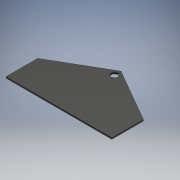
# Autodesk Inventor part: BA15
Saved by Autodesk Inventor 2017 (Build 210142000, 142)
## iProperties
Created: 2019-05-29
Part Number: BA15
Material: Wood (Cherry)
Document SubType Name: Modeling
Designer: Dell
Density: 0.63 g/cm^3
Appearance: Smooth - Black
Mass: 254.003 g
Surface Area: 1468.73 cm^2
Volume: 403.179 cm^3
Author: Dell
Autodesk Inventor part; units mm, degrees
ref_plane "YZ Plane" through (0, 0, 0) normal (1, 0, 0) x (0, 1, 0)
ref_plane "XZ Plane" through (0, 0, 0) normal (0, 1, 0) x (-1, 0, 0)
ref_plane "XY Plane" through (0, 0, 0) normal (0, 0, 1) x (1, 0, 0)
sketch "Sketch1" plane through (0, 0, 0) normal (0, 0, 1) x (1, 0, 0)
  line L0 (0, 0) -> (0, 201.9592)
  line L1 (0, 201.9592) -> (262.89, 353.7388)
  line L2 (262.89, 353.7388) -> (525.78, 201.9592)
  line L3 (525.78, 201.9592) -> (525.78, 0)
  line L4 (525.78, 0) -> (0, 0)
  point P0 (262.89, 0)
  dimension "d0" = 525.78
  dimension "d1" = 120
  dimension "d2" = 201.9592
  constraints: 10 end point, 1 horizontal alignment, 1 midpoint, 1 parallel, 1 perpendicular, 1 vertical, 1 vertical alignment
  measures "d0" distance of L3.end L0.start
  measures "d1" angle of L2 L1
  measures "d2" distance of L0.start L0.end
extrude "Extrusion1" add sketch "Sketch1" along normal blind 6.35
sketch "Sketch3" plane through (0, 0, 6.35) normal (0, 0, 1) x (1, 0, 0)
  line L0 (50.8, 180.4886) -> (474.98, 180.4886)
  line L1 (474.98, 180.4886) -> (474.98, 50.8)
  line L2 (474.98, 50.8) -> (50.8, 50.8)
  line L3 (50.8, 50.8) -> (50.8, 180.4886)
  line L4 (0, 201.9592) -> (0, 0) projected
  line L5 (50.8, 180.4886) -> (262.89, 302.9388)
  line L6 (262.89, 302.9388) -> (474.98, 180.4886)
  line L7 (525.78, 0) -> (0, 0) projected
  line L8 (0, 201.9592) -> (0, 0) projected
  line L9 (0, 0) -> (525.78, 0) projected
  line L10 (525.78, 0) -> (525.78, 201.9592) projected
  line L11 (525.78, 201.9592) -> (262.89, 353.7388) projected
  line L12 (262.89, 353.7388) -> (0, 201.9592) projected
  point P0 (262.89, 180.4886)
  dimension "d15" = 120
  dimension "d16" = 50.8
  dimension "d17" = 50.8
  dimension "d18" = 50.8
  constraints: 12 end point, 2 parallel, 2 vertical alignment, 1 horizontal, 1 midpoint, 1 perpendicular
  measures "d15" angle of L6 L5
  measures "d16" distance between parallel lines of L4 L3
  measures "d17" distance between parallel lines of L7 L2
  measures "d18" distance of point (262.89, 353.739) L5.end
extrude "Extrusion3" cut sketch "Sketch3" against normal through all
sketch "Sketch8" plane through (0, 0, 6.35) normal (0, 0, 1) x (1, 0, 0)
  line L0 (50.8, 50.8) -> (474.98, 50.8) projected
  line L1 (50.8, 180.4886) -> (50.8, 50.8) projected
  line L2 (50.8, 50.8) -> (474.98, 50.8) projected
  line L3 (474.98, 50.8) -> (474.98, 180.4886) projected
  line L4 (474.98, 180.4886) -> (262.89, 302.9388) projected
  line L5 (262.89, 302.9388) -> (50.8, 180.4886) projected
  line L6 (53.975, 178.6555) -> (53.975, 53.975)
  line L7 (53.975, 53.975) -> (471.805, 53.975)
  line L8 (471.805, 53.975) -> (471.805, 178.6555)
  line L9 (471.805, 178.6555) -> (262.89, 299.2727)
  line L10 (262.89, 299.2727) -> (53.975, 178.6555)
  point P0 (0, 0)
  dimension "d48" = 3.175
  constraints: 10 end point, 4 other
  measures "d48" distance between parallel lines of L5 L10
extrude "Extrusion8" cut sketch "Sketch8" against normal through all
sketch "Sketch9" plane through (0, 0, 6.35) normal (0, 0, 1) x (1, 0, 0)
  line L0 (262.89, 288.5374) -> (275.59, 281.205)
  line L1 (275.59, 281.205) -> (275.59, 266.5403)
  line L2 (275.59, 266.5403) -> (262.89, 259.208)
  line L3 (262.89, 259.208) -> (250.19, 266.5403)
  line L4 (250.19, 266.5403) -> (250.19, 281.205)
  line L5 (250.19, 281.205) -> (262.89, 288.5374)
  point P0 (0, 0)
  point P1 (262.89, 273.8727)
  point P2 (262.89, 299.2727)
  dimension "d51" = 25.4
  dimension "d52" = 25.4
  constraints: 12 end point, 2 vertical alignment, 13 other
  measures "d51" distance between parallel lines of L4 L1
  measures "d52" distance of point (262.89, 299.273) point (262.89, 273.873)
extrude "Extrusion9" cut sketch "Sketch9" against normal through all
equation "\"d3\" = Panel_Thickness"
equation "\"Panel_Thickness\" = 6.35"
equation "\"Fit_Tolerance\" = 1.27"
equation "\"Tool_Dia\" = 6.35"
body "Solid1"
